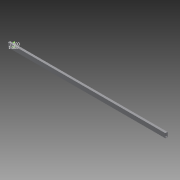
# Autodesk Inventor part: box beam
Saved by Autodesk Inventor 2015 (Build 190159000, 159)
## iProperties
Created: 2015-01-17
Part Number: box beam
Material: Generic
Document SubType Name: Modeling
Designer: whitaus15
Density: 1 g/cm^3
Appearance: Default
Author: whitaus15
Autodesk Inventor part; units mm, degrees
ref_plane "YZ Plane" through (0, 0, 0) normal (1, 0, 0) x (0, 1, 0)
ref_plane "XZ Plane" through (0, 0, 0) normal (0, 1, 0) x (-1, 0, 0)
ref_plane "XY Plane" through (0, 0, 0) normal (0, 0, 1) x (1, 0, 0)
sketch "Sketch1" plane through (0, 0, 0) normal (1, 0, 0) x (0, 1, 0)
  line L0 (9.5793, -16.837) -> (-41.2207, -16.837)
  line L1 (-41.2207, -16.837) -> (-41.2207, -42.237)
  line L2 (-41.2207, -42.237) -> (9.5793, -42.237)
  line L3 (9.5793, -42.237) -> (9.5793, -16.837)
  point P0 (0, 0)
  dimension "d0" = 50.8
  dimension "d1" = 25.4
  constraints: 8 end point, 2 parallel, 1 horizontal, 1 perpendicular
  measures "d0" distance of L2.end L1.end
  measures "d1" distance of L1.end L0.end
sketch "Sketch2" plane through (0, 0, 0) normal (1, 0, 0) x (0, 1, 0)
  point P0 (0, 0)
sketch "Sketch3" plane through (0, 0, 0) normal (1, 0, 0) x (0, 1, 0)
  line L0 (36.8031, 29.6629) -> (-6.3261, 29.6629)
  line L1 (-6.3261, 29.6629) -> (-6.3261, 11.9337)
  line L2 (-6.3261, 11.9337) -> (36.8031, 11.9337)
  line L3 (36.8031, 11.9337) -> (36.8031, 29.6629)
  line L4 (40.6385, 33.4983) -> (-10.1615, 33.4983)
  line L5 (-10.1615, 33.4983) -> (-10.1615, 8.0983)
  line L6 (-10.1615, 8.0983) -> (40.6385, 8.0983)
  line L7 (40.6385, 8.0983) -> (40.6385, 33.4983)
  point P0 (0, 0)
  dimension "d2" = 43.1292
  dimension "d3" = 17.7292
  dimension "d4" = 50.8
  dimension "d5" = 25.4
  dimension "d6" = 3.8354
  dimension "d7" = 3.8354
  constraints: 16 end point, 4 parallel, 2 horizontal, 2 perpendicular
  measures "d2" distance of L2.end L1.end
  measures "d3" distance of L1.end L0.end
  measures "d4" distance of L6.end L5.end
  measures "d5" distance of L5.end L4.end
  measures "d6" distance between parallel lines of L7 L3
  measures "d7" distance between parallel lines of L4 L0
extrude "Extrusion1" add sketch "Sketch3" along normal blind 1828.8
sketch "Sketch4" plane through (0, -10.1615, 33.4983) normal (0, 0, 1) x (1, 0, 0)
  circle A0 centre (25.4, 25.4) radius 14.2875
  line L0 (0, 50.8) -> (1828.8, 50.8) projected
  line L1 (0, 50.8) -> (0, 0) projected
  point P0 (0, 10.1615)
  dimension "d10" = 28.575
  dimension "d11" = 25.4
  dimension "d12" = 25.4
  constraints: 1 centre point
  measures "d10" diameter of A0
  measures "d11" distance from line of A0.centre L0
  measures "d12" distance from line of L1 A0.centre
hole "Hole1" at (25.4, 15.2385, 33.4983) direction (0, 0, -1) diameter 31.75 end through all
body "Solid1"
